Autodesk Inventor part; units mm, degrees
(part 2 of 2)
sketch "Sketch1" plane through (0, 0, 0) normal (0, 0, 1) x (1, 0, 0)
  arc A0 (17.4991, 1.1436) -> (17.4688, 1.3572) centre (17.3172, 1.2268) ccw
  arc A1 (17.4991, 1.1436) -> (17.4991, -1.1436) centre (20, 0) ccw
  arc A2 (8.5, -9.7678) -> (8.3536, -9.4142) centre (8, -9.7678) ccw
  line L0 (3.5858, -4.6464) -> (8.3536, -9.4142)
  arc A3 (3.5858, -4.6464) -> (3.2322, -4.5) centre (3.2322, -5) ccw
  line L1 (0.9536, -4.5) -> (3.2322, -4.5)
  arc A4 (0.8536, -4.4732) -> (0.9536, -4.5) centre (0.9536, -4.3) ccw
  line L2 (0.1, -4.0381) -> (0.8536, -4.4732)
  arc A5 (0.1, -4.0381) -> (-0.1, -4.0381) centre (0, -4.2113) ccw
  line L3 (-0.8536, -4.4732) -> (-0.1, -4.0381)
  arc A6 (-0.9536, -4.5) -> (-0.8536, -4.4732) centre (-0.9536, -4.3) ccw
  line L4 (-3.2322, -4.5) -> (-0.9536, -4.5)
  arc A7 (-3.2322, -4.5) -> (-3.5858, -4.6464) centre (-3.2322, -5) ccw
  line L5 (-3.5858, -4.6464) -> (-5.8536, -6.9142)
  arc A8 (-7.2678, -7.5) -> (-5.8536, -6.9142) centre (-7.2678, -5.5) ccw
  line L6 (-7.2678, -7.5) -> (-8, -7.5)
  arc A9 (-8, -7.5) -> (-8.5, -8) centre (-8, -8) ccw
  line L7 (-8.5, -12) -> (-8.5, -8)
  arc A10 (-8.5, -12) -> (-8, -12.5) centre (-8, -12) ccw
  line L8 (-7.2678, -12.5) -> (-8, -12.5)
  arc A11 (-5.8536, -13.0858) -> (-7.2678, -12.5) centre (-7.2678, -14.5) ccw
  line L9 (-3.5858, -15.3536) -> (-5.8536, -13.0858)
  arc A12 (-3.5858, -15.3536) -> (-3.2322, -15.5) centre (-3.2322, -15) ccw
  line L10 (-0.9536, -15.5) -> (-3.2322, -15.5)
  arc A13 (-0.8536, -15.5268) -> (-0.9536, -15.5) centre (-0.9536, -15.7) ccw
  line L11 (-0.1, -15.9619) -> (-0.8536, -15.5268)
  arc A14 (-0.1, -15.9619) -> (0.1, -15.9619) centre (0, -15.7887) ccw
  line L12 (0.8536, -15.5268) -> (0.1, -15.9619)
  arc A15 (0.9536, -15.5) -> (0.8536, -15.5268) centre (0.9536, -15.7) ccw
  line L13 (3.2322, -15.5) -> (0.9536, -15.5)
  arc A16 (3.2322, -15.5) -> (3.5858, -15.3536) centre (3.2322, -15) ccw
  line L14 (5.8536, -13.0858) -> (3.5858, -15.3536)
  arc A17 (7.2678, -12.5) -> (5.8536, -13.0858) centre (7.2678, -14.5) ccw
  line L15 (7.2678, -12.5) -> (8, -12.5)
  arc A18 (8, -12.5) -> (8.5, -12) centre (8, -12) ccw
  line L16 (2.5259, 1.3623) -> (2.8916, 1.8006)
  arc A19 (2.8916, 1.8006) -> (2.9015, 2.0439) centre (2.738, 1.9287) ccw
  arc A20 (2.9015, 2.0439) -> (2.0439, 2.9015) centre (0, 0) ccw
  arc A21 (2.0439, 2.9015) -> (1.8006, 2.8916) centre (1.9287, 2.738) ccw
  line L17 (1.3623, 2.5259) -> (1.8006, 2.8916)
  arc A22 (1.1505, 2.4978) -> (1.3623, 2.5259) centre (1.2342, 2.6794) ccw
  arc A23 (1.1505, 2.4978) -> (-1.1505, 2.4978) centre (0, 0) ccw
  arc A24 (-1.3623, 2.5259) -> (-1.1505, 2.4978) centre (-1.2342, 2.6794) ccw
  line L18 (-1.3623, 2.5259) -> (-1.8006, 2.8916)
  arc A25 (-1.8006, 2.8916) -> (-2.0439, 2.9015) centre (-1.9287, 2.738) ccw
  arc A26 (-2.0439, 2.9015) -> (-2.9015, 2.0439) centre (0, 0) ccw
  arc A27 (-2.9015, 2.0439) -> (-2.8912, 1.8002) centre (-2.738, 1.9287) ccw
  line L19 (-2.8912, 1.8002) -> (-2.5243, 1.3629)
  arc A28 (-2.4869, 1.1738) -> (-2.5243, 1.3629) centre (-2.6775, 1.2343) ccw
  arc A29 (-2.4869, 1.1738) -> (-2.4971, -1.152) centre (0, 0) ccw
  arc A30 (-2.5243, -1.3629) -> (-2.4971, -1.152) centre (-2.6787, -1.2357) ccw
  line L20 (-2.8912, -1.8002) -> (-2.5243, -1.3629)
  arc A31 (-2.8912, -1.8002) -> (-2.9015, -2.0439) centre (-2.738, -1.9287) ccw
  arc A32 (-2.9015, -2.0439) -> (-2.0359, -2.9071) centre (0, 0) ccw
  arc A33 (-2.0359, -2.9071) -> (-1.7927, -2.8965) centre (-1.9212, -2.7433) ccw
  line L21 (-1.7927, -2.8965) -> (-1.3554, -2.5296)
  arc A34 (-1.1436, -2.5009) -> (-1.3554, -2.5296) centre (-1.2268, -2.6828) ccw
  arc A35 (-1.1436, -2.5009) -> (1.1505, -2.4978) centre (0, 0) ccw
  arc A36 (1.3623, -2.5259) -> (1.1505, -2.4978) centre (1.2342, -2.6794) ccw
  line L22 (1.3623, -2.5259) -> (1.8006, -2.8916)
  arc A37 (1.8006, -2.8916) -> (2.0439, -2.9015) centre (1.9287, -2.738) ccw
  arc A38 (2.0439, -2.9015) -> (2.9015, -2.0439) centre (0, 0) ccw
  arc A39 (2.9015, -2.0439) -> (2.8916, -1.8006) centre (2.738, -1.9287) ccw
  line L23 (2.8916, -1.8006) -> (2.5259, -1.3623)
  arc A40 (2.4978, -1.1505) -> (2.5259, -1.3623) centre (2.6794, -1.2342) ccw
  arc A41 (2.4978, -1.1505) -> (2.4978, 1.1505) centre (0, 0) ccw
  line L24 (-1.3623, -17.4741) -> (-1.8006, -17.1084)
  arc A42 (-1.8006, -17.1084) -> (-2.0439, -17.0985) centre (-1.9287, -17.262) ccw
  arc A43 (-2.0439, -17.0985) -> (-2.9015, -17.9561) centre (0, -20) ccw
  arc A44 (-2.9015, -17.9561) -> (-2.8916, -18.1994) centre (-2.738, -18.0713) ccw
  line L25 (-2.8916, -18.1994) -> (-2.5259, -18.6377)
  arc A45 (-2.4978, -18.8495) -> (-2.5259, -18.6377) centre (-2.6794, -18.7658) ccw
  arc A46 (-2.4978, -18.8495) -> (-2.4978, -21.1505) centre (0, -20) ccw
  arc A47 (-2.5259, -21.3623) -> (-2.4978, -21.1505) centre (-2.6794, -21.2342) ccw
  line L26 (-2.8916, -21.8006) -> (-2.5259, -21.3623)
  arc A48 (-2.8916, -21.8006) -> (-2.9015, -22.0439) centre (-2.738, -21.9287) ccw
  arc A49 (-2.9015, -22.0439) -> (-2.0439, -22.9015) centre (0, -20) ccw
  arc A50 (-2.0439, -22.9015) -> (-1.8006, -22.8916) centre (-1.9287, -22.738) ccw
  line L27 (-1.8006, -22.8916) -> (-1.3623, -22.5259)
  arc A51 (-1.1505, -22.4978) -> (-1.3623, -22.5259) centre (-1.2342, -22.6794) ccw
  arc A52 (-1.1505, -22.4978) -> (1.1505, -22.4978) centre (0, -20) ccw
  arc A53 (1.3623, -22.5259) -> (1.1505, -22.4978) centre (1.2342, -22.6794) ccw
  line L28 (1.3623, -22.5259) -> (1.8006, -22.8916)
  arc A54 (1.8006, -22.8916) -> (2.0439, -22.9015) centre (1.9287, -22.738) ccw
  arc A55 (2.0439, -22.9015) -> (2.9015, -22.0439) centre (0, -20) ccw
  arc A56 (2.9015, -22.0439) -> (2.8916, -21.8006) centre (2.738, -21.9287) ccw
  line L29 (2.8916, -21.8006) -> (2.5259, -21.3623)
  arc A57 (2.4978, -21.1505) -> (2.5259, -21.3623) centre (2.6794, -21.2342) ccw
  arc A58 (2.4978, -21.1505) -> (2.4978, -18.8495) centre (0, -20) ccw
  arc A59 (2.5259, -18.6377) -> (2.4978, -18.8495) centre (2.6794, -18.7658) ccw
  arc A60 (-3.55, 9.8) -> (-3.75, 10) centre (-3.75, 9.8) ccw
  line L30 (12, 8.5) -> (8, 8.5)
  arc A61 (17.4688, -1.3572) -> (17.4991, -1.1436) centre (17.3172, -1.2268) ccw
  line L31 (8.5, -12) -> (8.5, -9.7678)
  arc A62 (2.5259, 1.3623) -> (2.4978, 1.1505) centre (2.6794, 1.2342) ccw
  arc A63 (-1.3623, -17.4741) -> (-1.1505, -17.5022) centre (-1.2342, -17.3206) ccw
  arc A64 (8, 8.5) -> (7.5, 8) centre (8, 8) ccw
  line L32 (7.5, 7.2678) -> (7.5, 8)
  arc A65 (6.9142, 5.8536) -> (7.5, 7.2678) centre (5.5, 7.2678) ccw
  line L33 (4.6464, 3.5858) -> (6.9142, 5.8536)
  arc A66 (4.6464, 3.5858) -> (4.5, 3.2322) centre (5, 3.2322) ccw
  line L34 (4.5, 0.9536) -> (4.5, 3.2322)
  arc A67 (4.4732, 0.8536) -> (4.5, 0.9536) centre (4.3, 0.9536) ccw
  line L35 (4.0381, 0.1) -> (4.4732, 0.8536)
  arc A68 (4.0381, 0.1) -> (4.0381, -0.1) centre (4.2113, 0) ccw
  line L36 (4.4732, -0.8536) -> (4.0381, -0.1)
  arc A69 (4.5, -0.9536) -> (4.4732, -0.8536) centre (4.3, -0.9536) ccw
  line L37 (4.5, -3.2322) -> (4.5, -0.9536)
  arc A70 (4.5, -3.2322) -> (4.6464, -3.5858) centre (5, -3.2322) ccw
  line L38 (9.4142, -8.3536) -> (4.6464, -3.5858)
  arc A71 (9.4142, -8.3536) -> (9.7678, -8.5) centre (9.7678, -8) ccw
  line L39 (12, -8.5) -> (9.7678, -8.5)
  arc A72 (12, -8.5) -> (12.5, -8) centre (12, -8) ccw
  line L40 (12.5, -7.2678) -> (12.5, -8)
  arc A73 (13.0858, -5.8536) -> (12.5, -7.2678) centre (14.5, -7.2678) ccw
  line L41 (13.0858, -5.8536) -> (15.3536, -3.5858)
  arc A74 (15.3536, -3.5858) -> (15.5, -3.2322) centre (15, -3.2322) ccw
  line L42 (15.5, -3.2322) -> (15.5, -0.9536)
  arc A75 (15.5268, -0.8536) -> (15.5, -0.9536) centre (15.7, -0.9536) ccw
  line L43 (15.5268, -0.8536) -> (15.9619, -0.1)
  arc A76 (15.9619, -0.1) -> (15.9619, 0.1) centre (15.7887, 0) ccw
  line L44 (15.9619, 0.1) -> (15.5268, 0.8536)
  arc A77 (15.5, 0.9536) -> (15.5268, 0.8536) centre (15.7, 0.9536) ccw
  line L45 (15.5, 0.9536) -> (15.5, 3.2322)
  arc A78 (15.5, 3.2322) -> (15.3536, 3.5858) centre (15, 3.2322) ccw
  line L46 (15.3536, 3.5858) -> (13.0858, 5.8536)
  arc A79 (12.5, 7.2678) -> (13.0858, 5.8536) centre (14.5, 7.2678) ccw
  line L47 (12.5, 7.2678) -> (12.5, 8)
  arc A80 (12.5, 8) -> (12, 8.5) centre (12, 8) ccw
  line L48 (17.1088, -1.8002) -> (17.4688, -1.3572)
  arc A81 (17.1088, -1.8002) -> (17.0985, -2.0439) centre (17.262, -1.9287) ccw
  arc A82 (17.0985, -2.0439) -> (17.9561, -2.9015) centre (20, 0) ccw
  arc A83 (17.9561, -2.9015) -> (18.1998, -2.8912) centre (18.0713, -2.738) ccw
  line L49 (18.1998, -2.8912) -> (18.6428, -2.5312)
  arc A84 (18.8564, -2.5009) -> (18.6428, -2.5312) centre (18.7732, -2.6828) ccw
  arc A85 (18.8564, -2.5009) -> (21.1436, -2.5009) centre (20, 0) ccw
  arc A86 (21.3554, -2.5296) -> (21.1436, -2.5009) centre (21.2268, -2.6828) ccw
  line L50 (21.7983, -2.8897) -> (21.3554, -2.5296)
  arc A87 (21.7983, -2.8897) -> (22.0439, -2.9015) centre (21.9287, -2.738) ccw
  arc A88 (22.0439, -2.9015) -> (22.9015, -2.0439) centre (20, 0) ccw
  arc A89 (22.9015, -2.0439) -> (22.8897, -1.7983) centre (22.738, -1.9287) ccw
  line L51 (22.5296, -1.3554) -> (22.8897, -1.7983)
  arc A90 (22.5009, -1.1436) -> (22.5296, -1.3554) centre (22.6828, -1.2268) ccw
  arc A91 (22.5009, -1.1436) -> (22.5009, 1.1436) centre (20, 0) ccw
  arc A92 (22.5296, 1.3554) -> (22.5009, 1.1436) centre (22.6828, 1.2268) ccw
  line L52 (22.5296, 1.3554) -> (22.8897, 1.7983)
  arc A93 (22.8897, 1.7983) -> (22.9015, 2.0439) centre (22.738, 1.9287) ccw
  arc A94 (22.9015, 2.0439) -> (22.0439, 2.9015) centre (20, 0) ccw
  arc A95 (22.0439, 2.9015) -> (21.7983, 2.8897) centre (21.9287, 2.738) ccw
  line L53 (21.3554, 2.5296) -> (21.7983, 2.8897)
  arc A96 (21.1436, 2.5009) -> (21.3554, 2.5296) centre (21.2268, 2.6828) ccw
  arc A97 (21.1436, 2.5009) -> (18.8564, 2.5009) centre (20, 0) ccw
  arc A98 (18.6428, 2.5312) -> (18.8564, 2.5009) centre (18.7732, 2.6828) ccw
  line L54 (18.1998, 2.8912) -> (18.6428, 2.5312)
  arc A99 (18.1998, 2.8912) -> (17.9561, 2.9015) centre (18.0713, 2.738) ccw
  arc A100 (17.9561, 2.9015) -> (17.0985, 2.0439) centre (20, 0) ccw
  arc A101 (17.0985, 2.0439) -> (17.1088, 1.8002) centre (17.262, 1.9287) ccw
  line L55 (17.4688, 1.3572) -> (17.1088, 1.8002)
  arc A102 (-9, 3) -> (-8.5, 3.5) centre (-9, 3.5) ccw
  line L56 (-9.3, 3) -> (-9, 3)
  arc A103 (-9.5, 3.2) -> (-9.3, 3) centre (-9.3, 3.2) ccw
  line L57 (-9.5, 3.2) -> (-9.5, 3.35)
  arc A104 (-9.5, 3.35) -> (-9.7, 3.55) centre (-9.7, 3.35) ccw
  line L58 (-9.8, 3.55) -> (-9.7, 3.55)
  arc A105 (-10, 3.75) -> (-9.8, 3.55) centre (-9.8, 3.75) ccw
  line L59 (-10, 3.75) -> (-10, 8.5)
  arc A106 (-8.5, 10) -> (-10, 8.5) centre (-8.5, 8.5) ccw
  line L60 (-8.5, 10) -> (-3.75, 10)
  line L61 (3.3, -29.5) -> (3.2, -29.5)
  arc A107 (3, -29.3) -> (3.2, -29.5) centre (3.2, -29.3) ccw
  line L62 (3, -29.3) -> (3, -29)
  arc A108 (3.5, -28.5) -> (3, -29) centre (3.5, -29) ccw
  line L63 (3.5, -28.5) -> (5.5, -28.5)
  arc A109 (5.5, -28.5) -> (6, -28) centre (5.5, -28) ccw
  line L64 (6, -28) -> (6, -27.2678)
  arc A110 (6, -27.2678) -> (5.8536, -26.9142) centre (5.5, -27.2678) ccw
  line L65 (5.8536, -26.9142) -> (3.5858, -24.6464)
  arc A111 (3.5858, -24.6464) -> (3.2322, -24.5) centre (3.2322, -25) ccw
  line L66 (3.2322, -24.5) -> (0.9536, -24.5)
  arc A112 (0.8536, -24.4732) -> (0.9536, -24.5) centre (0.9536, -24.3) ccw
  line L67 (0.8536, -24.4732) -> (0.1, -24.0381)
  arc A113 (0.1, -24.0381) -> (-0.1, -24.0381) centre (0, -24.2113) ccw
  line L68 (-0.8536, -24.4732) -> (-0.1, -24.0381)
  arc A114 (-0.9536, -24.5) -> (-0.8536, -24.4732) centre (-0.9536, -24.3) ccw
  line L69 (-0.9536, -24.5) -> (-3.2322, -24.5)
  arc A115 (-3.2322, -24.5) -> (-3.5858, -24.6464) centre (-3.2322, -25) ccw
  line L70 (-5.8536, -26.9142) -> (-3.5858, -24.6464)
  arc A116 (-5.8536, -26.9142) -> (-6, -27.2678) centre (-5.5, -27.2678) ccw
  line L71 (-6, -28) -> (-6, -27.2678)
  arc A117 (-6, -28) -> (-5.5, -28.5) centre (-5.5, -28) ccw
  line L72 (-5.5, -28.5) -> (-3.5, -28.5)
  arc A118 (-3, -29) -> (-3.5, -28.5) centre (-3.5, -29) ccw
  line L73 (-3, -29.3) -> (-3, -29)
  arc A119 (-3.2, -29.5) -> (-3, -29.3) centre (-3.2, -29.3) ccw
  line L74 (-3.2, -29.5) -> (-3.3, -29.5)
  arc A120 (-3.3, -29.5) -> (-3.5, -29.7) centre (-3.3, -29.7) ccw
  line L75 (-3.5, -29.8) -> (-3.5, -29.7)
  arc A121 (-3.7, -30) -> (-3.5, -29.8) centre (-3.7, -29.8) ccw
  line L76 (-3.7, -30) -> (-8.5, -30)
  arc A122 (-10, -28.5) -> (-8.5, -30) centre (-8.5, -28.5) ccw
  line L77 (-10, -28.5) -> (-10, -23.75)
  arc A123 (-9.8, -23.55) -> (-10, -23.75) centre (-9.8, -23.75) ccw
  line L78 (-9.8, -23.55) -> (-9.7, -23.55)
  arc A124 (-9.7, -23.55) -> (-9.5, -23.35) centre (-9.7, -23.35) ccw
  line L79 (-9.5, -23.35) -> (-9.5, -23.2)
  arc A125 (-9.3, -23) -> (-9.5, -23.2) centre (-9.3, -23.2) ccw
  line L80 (-9.3, -23) -> (-9, -23)
  arc A126 (-8.5, -23.5) -> (-9, -23) centre (-9, -23.5) ccw
  line L81 (-8.5, -23.5) -> (-8.5, -25.5)
  arc A127 (-8.5, -25.5) -> (-8, -26) centre (-8, -25.5) ccw
  line L82 (-8, -26) -> (-7.2678, -26)
  arc A128 (-7.2678, -26) -> (-6.9142, -25.8536) centre (-7.2678, -25.5) ccw
  line L83 (-6.9142, -25.8536) -> (-4.6464, -23.5858)
  arc A129 (-4.6464, -23.5858) -> (-4.5, -23.2322) centre (-5, -23.2322) ccw
  line L84 (-4.5, -23.2322) -> (-4.5, -20.9536)
  arc A130 (-4.4732, -20.8536) -> (-4.5, -20.9536) centre (-4.3, -20.9536) ccw
  line L85 (-4.4732, -20.8536) -> (-4.0381, -20.1)
  arc A131 (-4.0381, -20.1) -> (-4.0381, -19.9) centre (-4.2113, -20) ccw
  line L86 (-4.0381, -19.9) -> (-4.4732, -19.1464)
  arc A132 (-4.5, -19.0464) -> (-4.4732, -19.1464) centre (-4.3, -19.0464) ccw
  line L87 (-4.5, -19.0464) -> (-4.5, -16.7678)
  arc A133 (-4.5, -16.7678) -> (-4.6464, -16.4142) centre (-5, -16.7678) ccw
  line L88 (-4.6464, -16.4142) -> (-6.9142, -14.1464)
  arc A134 (-6.9142, -14.1464) -> (-7.2678, -14) centre (-7.2678, -14.5) ccw
  line L89 (-7.2678, -14) -> (-8, -14)
  arc A135 (-8, -14) -> (-8.5, -14.5) centre (-8, -14.5) ccw
  line L90 (-8.5, -16.5) -> (-8.5, -14.5)
  arc A136 (-9, -17) -> (-8.5, -16.5) centre (-9, -16.5) ccw
  line L91 (-9, -17) -> (-9.3, -17)
  arc A137 (-9.5, -16.8) -> (-9.3, -17) centre (-9.3, -16.8) ccw
  line L92 (-9.5, -16.8) -> (-9.5, -16.65)
  arc A138 (-9.5, -16.65) -> (-9.7, -16.45) centre (-9.7, -16.65) ccw
  line L93 (-9.7, -16.45) -> (-9.8, -16.45)
  arc A139 (-10, -16.25) -> (-9.8, -16.45) centre (-9.8, -16.25) ccw
  line L94 (-10, -16.25) -> (-10, -3.75)
  arc A140 (-9.8, -3.55) -> (-10, -3.75) centre (-9.8, -3.75) ccw
  line L95 (-9.7, -3.55) -> (-9.8, -3.55)
  arc A141 (-9.7, -3.55) -> (-9.5, -3.35) centre (-9.7, -3.35) ccw
  line L96 (-9.5, -3.35) -> (-9.5, -3.2)
  arc A142 (-9.3, -3) -> (-9.5, -3.2) centre (-9.3, -3.2) ccw
  line L97 (-9, -3) -> (-9.3, -3)
  arc A143 (-8.5, -3.5) -> (-9, -3) centre (-9, -3.5) ccw
  line L98 (-8.5, -5.5) -> (-8.5, -3.5)
  arc A144 (-8.5, -5.5) -> (-8, -6) centre (-8, -5.5) ccw
  line L99 (-7.2678, -6) -> (-8, -6)
  arc A145 (-7.2678, -6) -> (-6.9142, -5.8536) centre (-7.2678, -5.5) ccw
  line L100 (-6.9142, -5.8536) -> (-4.6464, -3.5858)
  arc A146 (-4.6464, -3.5858) -> (-4.5, -3.2322) centre (-5, -3.2322) ccw
  line L101 (-4.5, -3.2322) -> (-4.5, -0.9536)
  arc A147 (-4.4732, -0.8536) -> (-4.5, -0.9536) centre (-4.3, -0.9536) ccw
  line L102 (-4.4732, -0.8536) -> (-4.0381, -0.1)
  arc A148 (-4.0381, -0.1) -> (-4.0381, 0.1) centre (-4.2113, 0) ccw
  line L103 (-4.4732, 0.8536) -> (-4.0381, 0.1)
  arc A149 (-4.5, 0.9536) -> (-4.4732, 0.8536) centre (-4.3, 0.9536) ccw
  line L104 (-4.5, 0.9536) -> (-4.5, 3.2322)
  arc A150 (-4.5, 3.2322) -> (-4.6464, 3.5858) centre (-5, 3.2322) ccw
  line L105 (-6.9142, 5.8536) -> (-4.6464, 3.5858)
  arc A151 (-6.9142, 5.8536) -> (-7.2678, 6) centre (-7.2678, 5.5) ccw
  line L106 (-8, 6) -> (-7.2678, 6)
  arc A152 (-8, 6) -> (-8.5, 5.5) centre (-8, 5.5) ccw
  line L107 (-8.5, 3.5) -> (-8.5, 5.5)
  line L108 (24.0381, -0.1) -> (24.4732, -0.8536)
  arc A153 (24.5, -0.9536) -> (24.4732, -0.8536) centre (24.3, -0.9536) ccw
  line L109 (24.5, -3.2322) -> (24.5, -0.9536)
  arc A154 (24.5, -3.2322) -> (24.6464, -3.5858) centre (25, -3.2322) ccw
  line L110 (24.6464, -3.5858) -> (26.9142, -5.8536)
  arc A155 (26.9142, -5.8536) -> (27.2678, -6) centre (27.2678, -5.5) ccw
  line L111 (27.2678, -6) -> (28, -6)
  arc A156 (28, -6) -> (28.5, -5.5) centre (28, -5.5) ccw
  line L112 (28.5, -5.5) -> (28.5, -3.5)
  arc A157 (29, -3) -> (28.5, -3.5) centre (29, -3.5) ccw
  line L113 (29, -3) -> (29.3, -3)
  arc A158 (29.5, -3.2) -> (29.3, -3) centre (29.3, -3.2) ccw
  line L114 (29.5, -3.3) -> (29.5, -3.2)
  arc A159 (29.5, -3.3) -> (29.7, -3.5) centre (29.7, -3.3) ccw
  line L115 (29.7, -3.5) -> (29.8, -3.5)
  arc A160 (30, -3.7) -> (29.8, -3.5) centre (29.8, -3.7) ccw
  line L116 (30, -8.5) -> (30, -3.7)
  arc A161 (28.5, -10) -> (30, -8.5) centre (28.5, -8.5) ccw
  line L117 (23.7, -10) -> (28.5, -10)
  arc A162 (23.5, -9.8) -> (23.7, -10) centre (23.7, -9.8) ccw
  line L118 (23.5, -9.8) -> (23.5, -9.7)
  arc A163 (23.5, -9.7) -> (23.3, -9.5) centre (23.3, -9.7) ccw
  line L119 (23.2, -9.5) -> (23.3, -9.5)
  arc A164 (23, -9.3) -> (23.2, -9.5) centre (23.2, -9.3) ccw
  line L120 (23, -9.3) -> (23, -9)
  arc A165 (23.5, -8.5) -> (23, -9) centre (23.5, -9) ccw
  line L121 (23.5, -8.5) -> (25.5, -8.5)
  arc A166 (25.5, -8.5) -> (26, -8) centre (25.5, -8) ccw
  line L122 (26, -8) -> (26, -7.2678)
  arc A167 (26, -7.2678) -> (25.8536, -6.9142) centre (25.5, -7.2678) ccw
  line L123 (25.8536, -6.9142) -> (23.5858, -4.6464)
  arc A168 (23.5858, -4.6464) -> (23.2322, -4.5) centre (23.2322, -5) ccw
  line L124 (23.2322, -4.5) -> (20.9536, -4.5)
  arc A169 (20.8536, -4.4732) -> (20.9536, -4.5) centre (20.9536, -4.3) ccw
  line L125 (20.8536, -4.4732) -> (20.1, -4.0381)
  arc A170 (20.1, -4.0381) -> (19.9, -4.0381) centre (20, -4.2113) ccw
  line L126 (19.1464, -4.4732) -> (19.9, -4.0381)
  arc A171 (19.0464, -4.5) -> (19.1464, -4.4732) centre (19.0464, -4.3) ccw
  line L127 (19.0464, -4.5) -> (16.7678, -4.5)
  arc A172 (16.7678, -4.5) -> (16.4142, -4.6464) centre (16.7678, -5) ccw
  line L128 (14.1464, -6.9142) -> (16.4142, -4.6464)
  arc A173 (14.1464, -6.9142) -> (14, -7.2678) centre (14.5, -7.2678) ccw
  line L129 (14, -8) -> (14, -7.2678)
  arc A174 (14, -8) -> (14.5, -8.5) centre (14.5, -8) ccw
  line L130 (14.5, -8.5) -> (16.5, -8.5)
  arc A175 (17, -9) -> (16.5, -8.5) centre (16.5, -9) ccw
  line L131 (17, -9.3) -> (17, -9)
  arc A176 (16.8, -9.5) -> (17, -9.3) centre (16.8, -9.3) ccw
  line L132 (16.65, -9.5) -> (16.8, -9.5)
  arc A177 (16.65, -9.5) -> (16.45, -9.7) centre (16.65, -9.7) ccw
  line L133 (16.45, -9.8) -> (16.45, -9.7)
  arc A178 (16.25, -10) -> (16.45, -9.8) centre (16.25, -9.8) ccw
  line L134 (11.5, -10) -> (16.25, -10)
  arc A179 (11.5, -10) -> (10, -11.5) centre (11.5, -11.5) ccw
  line L135 (10, -16.3) -> (10, -11.5)
  arc A180 (9.8, -16.5) -> (10, -16.3) centre (9.8, -16.3) ccw
  line L136 (9.8, -16.5) -> (9.7, -16.5)
  arc A181 (9.7, -16.5) -> (9.5, -16.7) centre (9.7, -16.7) ccw
  line L137 (9.5, -16.8) -> (9.5, -16.7)
  arc A182 (9.3, -17) -> (9.5, -16.8) centre (9.3, -16.8) ccw
  line L138 (9.3, -17) -> (9, -17)
  arc A183 (8.5, -16.5) -> (9, -17) centre (9, -16.5) ccw
  line L139 (8.5, -16.5) -> (8.5, -14.5)
  arc A184 (8.5, -14.5) -> (8, -14) centre (8, -14.5) ccw
  line L140 (7.2678, -14) -> (8, -14)
  arc A185 (7.2678, -14) -> (6.9142, -14.1464) centre (7.2678, -14.5) ccw
  line L141 (4.6464, -16.4142) -> (6.9142, -14.1464)
  arc A186 (4.6464, -16.4142) -> (4.5, -16.7678) centre (5, -16.7678) ccw
  line L142 (4.5, -19.0464) -> (4.5, -16.7678)
  arc A187 (4.4732, -19.1464) -> (4.5, -19.0464) centre (4.3, -19.0464) ccw
  line L143 (4.0381, -19.9) -> (4.4732, -19.1464)
  arc A188 (4.0381, -19.9) -> (4.0381, -20.1) centre (4.2113, -20) ccw
  line L144 (4.0381, -20.1) -> (4.4732, -20.8536)
  arc A189 (4.5, -20.9536) -> (4.4732, -20.8536) centre (4.3, -20.9536) ccw
  line L145 (4.5, -23.2322) -> (4.5, -20.9536)
  arc A190 (4.5, -23.2322) -> (4.6464, -23.5858) centre (5, -23.2322) ccw
  line L146 (4.6464, -23.5858) -> (6.9142, -25.8536)
  arc A191 (6.9142, -25.8536) -> (7.2678, -26) centre (7.2678, -25.5) ccw
  line L147 (7.2678, -26) -> (8, -26)
  arc A192 (8, -26) -> (8.5, -25.5) centre (8, -25.5) ccw
  line L148 (8.5, -25.5) -> (8.5, -23.5)
  arc A193 (9, -23) -> (8.5, -23.5) centre (9, -23.5) ccw
  line L149 (9, -23) -> (9.3, -23)
  arc A194 (9.5, -23.2) -> (9.3, -23) centre (9.3, -23.2) ccw
  line L150 (9.5, -23.3) -> (9.5, -23.2)
  arc A195 (9.5, -23.3) -> (9.7, -23.5) centre (9.7, -23.3) ccw
  line L151 (9.7, -23.5) -> (9.8, -23.5)
  arc A196 (10, -23.7) -> (9.8, -23.5) centre (9.8, -23.7) ccw
  line L152 (10, -28.5) -> (10, -23.7)
  arc A197 (8.5, -30) -> (10, -28.5) centre (8.5, -28.5) ccw
  line L153 (8.5, -30) -> (3.7, -30)
  arc A198 (3.5, -29.8) -> (3.7, -30) centre (3.7, -29.8) ccw
  line L154 (3.5, -29.8) -> (3.5, -29.7)
  arc A199 (3.5, -29.7) -> (3.3, -29.5) centre (3.3, -29.7) ccw
  line L155 (2.5259, -18.6377) -> (2.8916, -18.1994)
  arc A200 (2.8916, -18.1994) -> (2.9015, -17.9561) centre (2.738, -18.0713) ccw
  arc A201 (2.9015, -17.9561) -> (2.0439, -17.0985) centre (0, -20) ccw
  arc A202 (2.0439, -17.0985) -> (1.8006, -17.1084) centre (1.9287, -17.262) ccw
  line L156 (1.3623, -17.4741) -> (1.8006, -17.1084)
  arc A203 (1.1505, -17.5022) -> (1.3623, -17.4741) centre (1.2342, -17.3206) ccw
  arc A204 (1.1505, -17.5022) -> (-1.1505, -17.5022) centre (0, -20) ccw
  line L157 (-3.55, 9.7) -> (-3.55, 9.8)
  arc A205 (-3.55, 9.7) -> (-3.35, 9.5) centre (-3.35, 9.7) ccw
  line L158 (-3.35, 9.5) -> (-3.2, 9.5)
  arc A206 (-3, 9.3) -> (-3.2, 9.5) centre (-3.2, 9.3) ccw
  line L159 (-3, 9) -> (-3, 9.3)
  arc A207 (-3.5, 8.5) -> (-3, 9) centre (-3.5, 9) ccw
  line L160 (-5.5, 8.5) -> (-3.5, 8.5)
  arc A208 (-5.5, 8.5) -> (-6, 8) centre (-5.5, 8) ccw
  line L161 (-6, 7.2678) -> (-6, 8)
  arc A209 (-6, 7.2678) -> (-5.8536, 6.9142) centre (-5.5, 7.2678) ccw
  line L162 (-3.5858, 4.6464) -> (-5.8536, 6.9142)
  arc A210 (-3.5858, 4.6464) -> (-3.2322, 4.5) centre (-3.2322, 5) ccw
  line L163 (-3.2322, 4.5) -> (-0.9536, 4.5)
  arc A211 (-0.8536, 4.4732) -> (-0.9536, 4.5) centre (-0.9536, 4.3) ccw
  line L164 (-0.8536, 4.4732) -> (-0.1, 4.0381)
  arc A212 (-0.1, 4.0381) -> (0.1, 4.0381) centre (0, 4.2113) ccw
  line L165 (0.1, 4.0381) -> (0.8536, 4.4732)
  arc A213 (0.9536, 4.5) -> (0.8536, 4.4732) centre (0.9536, 4.3) ccw
  line L166 (0.9536, 4.5) -> (3.2322, 4.5)
  arc A214 (3.2322, 4.5) -> (3.5858, 4.6464) centre (3.2322, 5) ccw
  line L167 (3.5858, 4.6464) -> (5.8536, 6.9142)
  arc A215 (5.8536, 6.9142) -> (6, 7.2678) centre (5.5, 7.2678) ccw
  line L168 (6, 7.2678) -> (6, 8)
  arc A216 (6, 8) -> (5.5, 8.5) centre (5.5, 8) ccw
  line L169 (5.5, 8.5) -> (3.5, 8.5)
  arc A217 (3, 9) -> (3.5, 8.5) centre (3.5, 9) ccw
  line L170 (3, 9) -> (3, 9.3)
  arc A218 (3.2, 9.5) -> (3, 9.3) centre (3.2, 9.3) ccw
  line L171 (3.2, 9.5) -> (3.3, 9.5)
  arc A219 (3.3, 9.5) -> (3.5, 9.7) centre (3.3, 9.7) ccw
  line L172 (3.5, 9.7) -> (3.5, 9.8)
  arc A220 (3.7, 10) -> (3.5, 9.8) centre (3.7, 9.8) ccw
  line L173 (3.7, 10) -> (16.2, 10)
  arc A221 (16.4, 9.8) -> (16.2, 10) centre (16.2, 9.8) ccw
  line L174 (16.4, 9.7) -> (16.4, 9.8)
  arc A222 (16.4, 9.7) -> (16.6, 9.5) centre (16.6, 9.7) ccw
  line L175 (16.6, 9.5) -> (16.8, 9.5)
  arc A223 (17, 9.3) -> (16.8, 9.5) centre (16.8, 9.3) ccw
  line L176 (17, 9) -> (17, 9.3)
  arc A224 (16.5, 8.5) -> (17, 9) centre (16.5, 9) ccw
  line L177 (14.5, 8.5) -> (16.5, 8.5)
  arc A225 (14.5, 8.5) -> (14, 8) centre (14.5, 8) ccw
  line L178 (14, 7.2678) -> (14, 8)
  arc A226 (14, 7.2678) -> (14.1464, 6.9142) centre (14.5, 7.2678) ccw
  line L179 (14.1464, 6.9142) -> (16.4142, 4.6464)
  arc A227 (16.4142, 4.6464) -> (16.7678, 4.5) centre (16.7678, 5) ccw
  line L180 (16.7678, 4.5) -> (19.0464, 4.5)
  arc A228 (19.1464, 4.4732) -> (19.0464, 4.5) centre (19.0464, 4.3) ccw
  line L181 (19.1464, 4.4732) -> (19.9, 4.0381)
  arc A229 (19.9, 4.0381) -> (20.1, 4.0381) centre (20, 4.2113) ccw
  line L182 (20.1, 4.0381) -> (20.8536, 4.4732)
  arc A230 (20.9536, 4.5) -> (20.8536, 4.4732) centre (20.9536, 4.3) ccw
  line L183 (20.9536, 4.5) -> (23.2322, 4.5)
  arc A231 (23.2322, 4.5) -> (23.5858, 4.6464) centre (23.2322, 5) ccw
  line L184 (23.5858, 4.6464) -> (25.8536, 6.9142)
  arc A232 (25.8536, 6.9142) -> (26, 7.2678) centre (25.5, 7.2678) ccw
  line L185 (26, 7.2678) -> (26, 8)
  arc A233 (26, 8) -> (25.5, 8.5) centre (25.5, 8) ccw
  line L186 (25.5, 8.5) -> (23.5, 8.5)
  arc A234 (23, 9) -> (23.5, 8.5) centre (23.5, 9) ccw
  line L187 (23, 9) -> (23, 9.3)
  arc A235 (23.2, 9.5) -> (23, 9.3) centre (23.2, 9.3) ccw
  line L188 (23.2, 9.5) -> (23.3, 9.5)
  arc A236 (23.3, 9.5) -> (23.5, 9.7) centre (23.3, 9.7) ccw
  line L189 (23.5, 9.7) -> (23.5, 9.8)
  arc A237 (23.7, 10) -> (23.5, 9.8) centre (23.7, 9.8) ccw
  line L190 (23.7, 10) -> (28.5, 10)
  arc A238 (30, 8.5) -> (28.5, 10) centre (28.5, 8.5) ccw
  line L191 (30, 3.7) -> (30, 8.5)
  arc A239 (29.8, 3.5) -> (30, 3.7) centre (29.8, 3.7) ccw
  line L192 (29.7, 3.5) -> (29.8, 3.5)
  arc A240 (29.7, 3.5) -> (29.5, 3.3) centre (29.7, 3.3) ccw
  line L193 (29.5, 3.2) -> (29.5, 3.3)
  arc A241 (29.3, 3) -> (29.5, 3.2) centre (29.3, 3.2) ccw
  line L194 (29, 3) -> (29.3, 3)
  arc A242 (28.5, 3.5) -> (29, 3) centre (29, 3.5) ccw
  line L195 (28.5, 3.5) -> (28.5, 5.5)
  arc A243 (28.5, 5.5) -> (28, 6) centre (28, 5.5) ccw
  line L196 (27.2678, 6) -> (28, 6)
  arc A244 (27.2678, 6) -> (26.9142, 5.8536) centre (27.2678, 5.5) ccw
  line L197 (24.6464, 3.5858) -> (26.9142, 5.8536)
  arc A245 (24.6464, 3.5858) -> (24.5, 3.2322) centre (25, 3.2322) ccw
  line L198 (24.5, 0.9536) -> (24.5, 3.2322)
  arc A246 (24.4732, 0.8536) -> (24.5, 0.9536) centre (24.3, 0.9536) ccw
  line L199 (24.0381, 0.1) -> (24.4732, 0.8536)
  arc A247 (24.0381, 0.1) -> (24.0381, -0.1) centre (24.2113, 0) ccw
  point P0 (0, 0)
  constraints: 1 other
extrude "Extrusion3" add sketch "Sketch1" along normal blind 10
body "Solid2"
